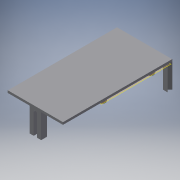
# Autodesk Inventor part: bottom
Saved by Autodesk Inventor 2018 (Build 220112000, 112)
## iProperties
Created: 2018-06-29
Part Number: bottom
Material: Generic
Document SubType Name: Modeling
Designer: erwin
Density: 1 g/cm^3
Appearance: Default
Author: erwin
Autodesk Inventor part; units mm, degrees
ref_plane "YZ Plane" through (0, 0, 0) normal (1, 0, 0) x (0, 1, 0)
ref_plane "XZ Plane" through (0, 0, 0) normal (0, 1, 0) x (-1, 0, 0)
ref_plane "XY Plane" through (0, 0, 0) normal (0, 0, 1) x (1, 0, 0)
ref_plane "Work Plane1" through (0, 0, 3) normal (0, 0, 1) x (1, 0, 0)
sketch "Sketch1" plane through (0, 0, 3) normal (0, 0, 1) x (1, 0, 0)
  circle A0 centre (-20, -24.5) radius 1.5 projected
  circle A1 centre (20, 17.5) radius 1.5 projected
  circle A2 centre (-20, 17.5) radius 1.5 projected
  circle A3 centre (20, -24.5) radius 1.5 projected
  line L0 (23, 27.5) -> (-23, 27.5) projected
  line L1 (-23, 27.5) -> (-23, -27.5) projected
  line L2 (-23, -27.5) -> (23, -27.5) projected
  line L3 (23, -27.5) -> (23, 27.5) projected
  line L4 (-16.6, 27.5) -> (17.4, 27.5) projected
  line L5 (17.4, 32.5) -> (17.4, 27.5) projected
  line L6 (-16.6, 32.5) -> (17.4, 32.5) projected
  line L7 (-16.6, 27.5) -> (-16.6, 32.5) projected
  line L8 (24, 32.5) -> (-24, 32.5)
  line L9 (-24, 32.5) -> (-24, -62.5)
  line L10 (-24, -62.5) -> (24, -62.5)
  line L11 (24, -62.5) -> (24, 32.5)
  point P0 (0, 0)
  dimension "d0" = 1
  dimension "d1" = 1
  dimension "d2" = 35
  constraints: 8 end point, 2 parallel, 1 horizontal, 1 perpendicular
  measures "d0" distance between parallel lines of L11 L3
  measures "d1" distance between parallel lines of L1 L9
  measures "d2" distance between parallel lines of L10 L2
extrude "Extrusion1" add sketch "Sketch1" along normal blind 2 contours A0 | A1 | A2 | A3 | L3 L2 L1 L0 | L0 L5 L8 L11 L10 L9 L7 L1 L2 L3 | L0 L7 L6 L5
sketch "Sketch2" plane through (0, 0, 3) normal (0, 0, -1) x (-1, 0, 0)
  circle A0 centre (20, -24.5) radius 1.5 projected
  circle A1 centre (-20, 17.5) radius 1.5 projected
  circle A2 centre (20, 17.5) radius 1.5 projected
  circle A3 centre (-20, -24.5) radius 1.5 projected
  line L0 (-17.4, 10.5) -> (-17.4, 27.5) projected
  line L1 (-17.4, 27.5) -> (-23, 27.5) projected
  line L2 (-23, 27.5) -> (-23, -27.5) projected
  line L3 (-23, -27.5) -> (23, -27.5) projected
  line L4 (23, -27.5) -> (23, 27.5) projected
  line L5 (23, 27.5) -> (16.6, 27.5) projected
  line L6 (16.6, 27.5) -> (16.6, 10.5) projected
  line L7 (16.6, 10.5) -> (-17.4, 10.5) projected
  circle A4 centre (20, 17.5) radius 3
  circle A5 centre (20, -24.5) radius 3
  circle A6 centre (-20, 17.5) radius 3
  circle A7 centre (-20, -24.5) radius 3
  point P0 (0, 0)
  dimension "d5" = 6
  dimension "d6" = 6
  dimension "d7" = 6
  dimension "d8" = 6
  constraints: 4 centre point, 4 coincident
  measures "d5" diameter of A4
  measures "d6" diameter of A5
  measures "d7" diameter of A6
  measures "d8" diameter of A7
extrude "Extrusion2" add sketch "Sketch2" along normal blind 3 contours A0 | A1 | A2 | A3 | A4 | A6 L0 | L0 A6 | A7 | A5
hole "Hole1" at (-20, 17.5, 0) direction (0, 0, 1) diameter 2 depth 4 tip angle 118
hole "Hole2" at (-20, -24.5, 0) direction (0, 0, 1) diameter 2 depth 4 tip angle 118
hole "Hole3" at (20, -24.5, 0) direction (0, 0, 1) diameter 2 depth 4 tip angle 118
hole "Hole4" at (20, 17.5, 0) direction (0, 0, 1) diameter 2 depth 4 tip angle 118
sketch "Sketch3" plane through (0, 0, 3) normal (0, 0, -1) x (-1, 0, 0)
  circle A0 centre (20, -24.5) radius 1.5 projected
  circle A1 centre (-20, 17.5) radius 1.5 projected
  circle A2 centre (20, 17.5) radius 1.5 projected
  circle A3 centre (-20, -24.5) radius 1.5 projected
  line L0 (-17.4, 10.5) -> (-17.4, 27.5) projected
  line L1 (-17.4, 27.5) -> (-23, 27.5) projected
  line L2 (-23, 27.5) -> (-23, -27.5) projected
  line L3 (-23, -27.5) -> (23, -27.5) projected
  line L4 (23, -27.5) -> (23, 27.5) projected
  line L5 (23, 27.5) -> (16.6, 27.5) projected
  line L6 (16.6, 27.5) -> (16.6, 10.5) projected
  line L7 (16.6, 10.5) -> (-17.4, 10.5) projected
  line L8 (-24, 32.5) -> (24, 32.5) projected
  line L9 (-24, 32.5) -> (-20, 32.5)
  line L10 (-20, 32.5) -> (-20, 28.5)
  line L11 (-20, 28.5) -> (-24, 28.5)
  line L12 (-24, 32.5) -> (24, 32.5) projected
  line L13 (-24, 32.5) -> (-22, 30.5)
  line L14 (-22, 30.5) -> (-24, 28.5)
  line L15 (-24, -62.5) -> (-24, 32.5) projected
  point P0 (0, 0)
  dimension "d56" = 4
  dimension "d57" = 90
  dimension "d58" = 4
  dimension "d59" = 4
  constraints: 10 end point, 2 perpendicular, 1 horizontal, 1 parallel
  measures "d56" distance of L9.end L10.end
  measures "d57" angle of L13 L14
  measures "d58" distance between parallel lines of L15 L10
  measures "d59" distance of L10.end L11.end
sketch "Sketch4" plane through (0, 0, 3) normal (0, 0, 1) x (1, 0, 0)
  point P0 (0, 0)
extrude "Extrusion3" add sketch "Sketch3" along normal blind 21 contours L8 L10 L11 L14 L13
mirror "Mirror1" about plane through (0, 0, 0) normal (1, 0, 0) of "Extrusion3"
sketch "Sketch5" plane through (0, 0, 3) normal (0, 0, -1) x (-1, 0, 0)
  line L0 (1.5, -68.6041) -> (-1.5, -68.6041)
  line L1 (-1.5, -68.6041) -> (-1.5, -56.3959)
  line L2 (-1.5, -56.3959) -> (1.5, -56.3959)
  line L3 (1.5, -56.3959) -> (1.5, -68.6041)
  line L4 (24, -62.5) -> (-24, -62.5) projected
  line L5 (1.5, -68.6041) -> (-1.5, -56.3959) construction
  line L6 (-1.5, -68.6041) -> (1.5, -56.3959) construction
  line L7 (5, -67.5) -> (-5, -67.5)
  line L8 (-5, -67.5) -> (-5, -57.5)
  line L9 (-5, -57.5) -> (5, -57.5)
  line L10 (5, -57.5) -> (5, -67.5)
  line L11 (5, -67.5) -> (-5, -57.5) construction
  line L12 (-5, -67.5) -> (5, -57.5) construction
  line L13 (5, -57.5) -> (-5, -57.5)
  line L14 (-5, -57.5) -> (-5, -62.5)
  line L15 (-5, -62.5) -> (5, -62.5)
  line L16 (5, -62.5) -> (5, -57.5)
  point P0 (0, 0)
  point P1 (0, -62.5)
  dimension "d62" = 3
  dimension "d63" = 10
  dimension "d64" = 10
  constraints: 32 end point, 6 midpoint, 6 parallel, 3 horizontal, 3 perpendicular
  measures "d62" distance of L1.end L2.end
  measures "d63" distance of L8.end L9.end
  measures "d64" distance of L7.end L8.end
extrude "Extrusion4" add sketch "Sketch5" along normal up to surface (21 mm away) contours L4 L1 L9 L3 | L3 L9 L10 L4 | L4 L8 L9 L1
sketch "Sketch6" plane through (-5, -57.5, 3) normal (0, 1, 0) x (1, 0, 0)
  circle A0 centre (5, 3) radius 1.5
  line L0 (3.5, 3) -> (3.5, 21)
  line L1 (10, 21) -> (0, 21) projected
  line L2 (6.5, 3) -> (6.5, 21)
  line L3 (6.5, 21) -> (3.5, 21)
  dimension "d67" = 3
  constraints: 6 end point, 2 point on circle, 2 vertical, 1 centre point, 1 coincident, 1 perpendicular, 1 point on line
  measures "d67" diameter of A0
extrude "Extrusion5" cut sketch "Sketch6" against normal blind 21
equation "\"d59\" = d58"
body "Solid1"
